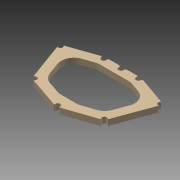
# Autodesk Inventor part: section1
Saved by Autodesk Inventor 2015 (Build 190159000, 159)
## iProperties
Created: 2017-09-23
Part Number: section1
Material: Polyethylene, High Density
Document SubType Name: Modeling
Designer: Mimoja
Density: 0.952 g/cm^3
Appearance: Smooth - Off-White
Mass: 359.919 g
Surface Area: 698.2 cm^2
Volume: 378.066 cm^3
Author: Mimoja
Autodesk Inventor part; units mm, degrees
ref_plane "YZ Plane" through (0, 0, 0) normal (1, 0, 0) x (0, 1, 0)
ref_plane "XZ Plane" through (0, 0, 0) normal (0, 1, 0) x (-1, 0, 0)
ref_plane "XY Plane" through (0, 0, 0) normal (0, 0, 1) x (1, 0, 0)
sketch "Sketch1" plane through (0, 0, 0) normal (0, 0, 1) x (1, 0, 0)
  line L0 (0, 19.2024) -> (-112.776, 57.6072)
  line L1 (-112.776, 57.6072) -> (-161.8488, 191.7192)
  line L2 (-161.8488, 191.7192) -> (-55.7784, 228.6)
  line L3 (0, 569.8709) -> (0, -138.2601) construction
  line L4 (-55.7784, 228.6) -> (0, 228.6)
  line L5 (0, 228.6) -> (0, 19.2024)
  point P0 (0, 0)
  dimension "d9" = 228.6
  dimension "d11" = 161.8488
  dimension "d15" = 191.7192
  dimension "d20" = 112.776
  dimension "d22" = 57.6072
  dimension "d39" = 55.7784
  dimension "d41" = 0
  dimension "d42" = 19.2024
  constraints: 12 end point, 1 collinear, 1 perpendicular, 1 point on line, 1 vertical
  measures "d9" vertical distance of point (0, 0) L2.end
  measures "d11" horizontal distance of point (0, 0) L1.end
  measures "d15" vertical distance of point (0, 0) L1.end
  measures "d20" horizontal distance of point (0, 0) L0.end
  measures "d22" vertical distance of point (0, 0) L0.end
  measures "d39" horizontal distance of point (0, 0) L2.end
  measures "d41" horizontal distance of point (0, 0) L0.start
  measures "d42" distance of point (0, 0) L0.start
extrude "Extrusion4" add sketch "Sketch1" along normal blind 18
hole "Hole2" at (0.0182, 221.5256, 18) direction (0, 0, -1) diameter 15 end through all
hole "Hole3" at (-155.5559, 188.7708, 18) direction (0, 0, -1) diameter 15 end through all
hole "Hole4" at (-108.5183, 61.8571, 18) direction (0, 0, -1) diameter 15 end through all
hole "Hole5" at (0.2097, 25.829, 18) direction (0, 0, -1) diameter 15 end through all
hole "Hole6" at (-53.869, 221.9476, 18) direction (0, 0, -1) diameter 15 end through all
fillet "Fillet6" radius 5.5 1 edges at (-2.4724, 228.6, 9)
fillet "Fillet7" radius 4 2 edges at (-50.4055, 228.6, 9) (-58.8915, 227.5176, 9)
fillet "Fillet8" radius 1 2 edges at (-158.2021, 181.7531, 9) (-151.747, 195.2316, 9)
fillet "Fillet9" radius 1 2 edges at (-115.412, 64.8112, 9) (-105.3263, 55.0703, 9)
fillet "Fillet10" radius 2 1 edges at (-5.6265, 21.1185, 9)
sketch "Sketch4" plane through (0, 0, 18) normal (0, 0, 1) x (1, 0, 0)
  line L0 (0, 33.326) -> (0, 214.0256) projected
  line L1 (0, 200.6) -> (-51.0494, 200.6)
  line L2 (-51.0494, 200.6) -> (-125.7756, 174.6176)
  line L3 (-125.7756, 174.6176) -> (-91.0802, 79.7979)
  line L4 (-91.0802, 79.7979) -> (-30, 58.9976)
  line L5 (-30, 58.9976) -> (0, 58.9976)
  line L6 (0, 200.6) -> (0, 58.9976)
  line L7 (-66.647, 224.821) -> (-149.9922, 195.8417) projected
  line L8 (-12.8861, 228.6) -> (-42.6791, 228.6) projected
  line L9 (-157.5584, 179.994) -> (-116.1314, 66.7773) projected
  line L10 (-103.3707, 54.4043) -> (-9.8336, 22.5511) projected
  point P0 (0, 0)
  point P1 (-15, 58.9976)
  dimension "d172" = 28
  dimension "d173" = 28
  dimension "d174" = 28
  dimension "d175" = 28
  dimension "d176" = 30
  constraints: 12 end point, 4 parallel, 2 horizontal, 2 point on line, 1 collinear, 1 midpoint
  measures "d172" distance between parallel lines of L7 L2
  measures "d173" distance between parallel lines of L8 L1
  measures "d174" distance between parallel lines of L9 L3
  measures "d175" distance between parallel lines of L10 L4
  measures "d176" distance of L4.end L5.end
extrude "Extrusion5" cut sketch "Sketch4" against normal through all
fillet "Fillet11" radius 40 4 edges at (-51.0494, 200.6, 9) (-125.7756, 174.6176, 9) (-91.0802, 79.7979, 9) (-30, 58.9976, 9)
mirror "Mirror3" about plane through (0, 0, 0) normal (1, 0, 0)
body "Solid4"
